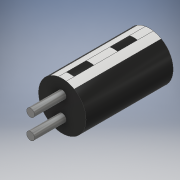
# Autodesk Inventor part: Kondensator
Saved by Autodesk Inventor 2017 SP1 (Build 210196100, 196)
## iProperties
Part Number: Kondensator
Material: Generisch
Document SubType Name: Modeling
Designer: Alex
Density: 1 g/cm^3
Appearance: Vorgabe
Durchmesser: 6.000 mm
Höhe: 11.000 mm
Author: Alex
Autodesk Inventor part; units mm, degrees
sketch "Skizze3" plane through (0, 0, 0) normal (0, 1, 0) x (-1, 0, 0)
  circle A0 centre (0, 0) radius 3
  dimension "Durchmesser" = 6
  constraints: 1 centre point, 1 coincident
  measures "Durchmesser" diameter of A0
extrude "Extrusion2" add sketch "Skizze3" along normal blind 11
sketch "Skizze4" plane through (0, 0, 0) normal (0, -1, 0) x (1, 0, 0)
  circle A0 centre (0, 1.27) radius 0.5
  circle A1 centre (0, -1.27) radius 0.5
  point P0 (0, 0)
  dimension "d6" = 1
  dimension "d7" = 1
  dimension "BeinAbstand" = 2.54
  dimension "BeinZuMitte" = 1.27
  constraints: 2 centre point, 2 vertical alignment
  measures "d6" diameter of A0
  measures "d7" diameter of A1
  measures "BeinAbstand" distance of A0.centre A1.centre
  measures "BeinZuMitte" distance of point (0, 0) A1.centre
extrude "Extrusion3" add sketch "Skizze4" along normal blind 4
ref_plane "Arbeitsebene1" through (-1.5, 0, 0) normal (1, 0, 0) x (0, 1, 0)
ref_plane "Arbeitsebene2" through (1.5, 0, 0) normal (1, 0, 0) x (0, 1, 0)
split_face "Trennen1"
split_face "Trennen2"
ref_plane "Arbeitsebene3" through (-0.5, 0, 0) normal (1, 0, 0) x (0, 1, 0)
ref_plane "Arbeitsebene4" through (0.5, 0, 0) normal (1, 0, 0) x (0, 1, 0)
ref_plane "Arbeitsebene5" through (0, 9, 0) normal (0, 1, 0) x (1, 0, 0)
ref_plane "Arbeitsebene6" through (0, 6.5, 0) normal (0, 1, 0) x (1, 0, 0)
sketch "Skizze5" plane through (0, 11, 0) normal (0, 1, 0) x (1, 0, 0)
  circle A0 centre (0, 0) radius 2.25
  dimension "d21" = 4.5
  constraints: 1 centre point, 1 coincident
  measures "d21" diameter of A0
extrude "Extrusion4" cut sketch "Skizze5" against normal blind 0.1
split_face "Trennen3"
split_face "Trennen4"
split_face "Trennen7"
split_face "Trennen8"
ref_plane "Arbeitsebene9" through (0, 3.5, 0) normal (0, -1, 0) x (1, 0, 0)
ref_plane "Arbeitsebene10" through (0, 1, 0) normal (0, -1, 0) x (1, 0, 0)
split_face "Trennen9"
split_face "Trennen10"
sketch "Skizze6" plane through (0, 10.9, 0) normal (0, 1, 0) x (1, 0, 0)
  line L0 (1.5, -0.025) -> (0, -0.025)
  line L1 (0, -0.025) -> (0, 0.025)
  line L2 (0, 0.025) -> (1.5, 0.025)
  line L3 (1.5, 0.025) -> (1.5, -0.025)
  line L4 (0.025, 1.5) -> (0.025, 0)
  line L5 (-0.025, 0) -> (-0.025, 1.5)
  line L6 (0.025, 0) -> (-0.025, 0)
  line L7 (-0.025, 1.5) -> (0.025, 1.5)
  line L8 (-1.5, 0.025) -> (0, 0.025)
  line L9 (0, -0.025) -> (-1.5, -0.025)
  line L10 (0, 0.025) -> (0, -0.025)
  line L11 (-1.5, -0.025) -> (-1.5, 0.025)
  line L12 (-0.025, -1.5) -> (-0.025, 0)
  line L13 (0.025, 0) -> (0.025, -1.5)
  line L14 (-0.025, 0) -> (0.025, 0)
  line L15 (0.025, -1.5) -> (-0.025, -1.5)
  point P0 (0, 0)
  point P1 (0, 0)
  point P2 (0, 0)
  point P3 (0, 0)
  dimension "d26" = 0.05
  dimension "d27" = 0.025
  dimension "d28" = 1.5
  dimension "d31" = 360
  constraints: 32 end point, 4 midpoint, 2 coincident, 2 parallel, 1 horizontal, 1 perpendicular, 35 other
  measures "d26" distance of L0.end L1.end
  measures "d27" distance from line of point (0, 0) L2
  measures "d28" distance of L1.end L2.end
extrude "Extrusion5" cut sketch "Skizze6" against normal blind 0.05
chamfer "Fase1" distance 0.05 angle 45 12 edges at (-0.025, 10.9, 0.7625) (0, 10.9, 1.5) (0.025, 10.9, 0.7625) (-0.7625, 10.9, 0.025) (-0.7625, 10.9, -0.025) (-0.025, 10.9, -0.7625) (0.025, 10.9, -0.7625) (0.7625, 10.9, 0.025) (0.7625, 10.9, -0.025) (0, 10.9, -1.5) (-1.5, 10.9, 0) (1.5, 10.9, 0)
fillet_without_effect "Rundung1"
equation "\"BeinZuMitte\" = 0.5 * BeinAbstand"
